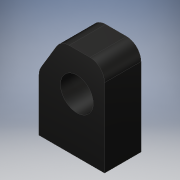
# Autodesk Inventor part: PilierCentral
Saved by Autodesk Inventor 2019 (Build 230136000, 136)
## iProperties
Created: 2019-07-30
Part Number: PilierCentral
Material: Plastique ABS
Document SubType Name: Modeling
Designer: Sébastien DI MERCURIO
Mass: 4.5474 g
Surface Area: 16.8462 cm^2
Volume: 4.29 cm^3
Density: 1.06 g/cm^3
Appearance: Lustré - Noir
Author: Sébastien DI MERCURIO
Autodesk Inventor part; units mm, degrees
ref_plane "YZ Plane" through (0, 0, 0) normal (1, 0, 0) x (0, 1, 0)
ref_plane "XZ Plane" through (0, 0, 0) normal (0, 1, 0) x (-1, 0, 0)
ref_plane "XY Plane" through (0, 0, 0) normal (0, 0, 1) x (1, 0, 0)
sketch "Esquisse1" plane through (0, 0, 0) normal (0, 0, 1) x (1, 0, 0)
  line L0 (0, 0) -> (0, 25.5)
  line L1 (0, 25.5) -> (-12, 25.5)
  line L2 (-12, 25.5) -> (-18, 15.5)
  line L3 (-18, 15.5) -> (-18, 0)
  line L4 (-18, 0) -> (0, 0)
  dimension "d0" = 18
  dimension "d1" = 25.5
  dimension "d2" = 15.5
  dimension "d3" = 12
  constraints: 10 end point, 2 perpendicular, 1 parallel, 1 vertical
  measures "d0" distance between parallel lines of L0 L3
  measures "d1" distance between parallel lines of L4 L1
  measures "d2" distance of L3.end L2.end
  measures "d3" distance of L0.end L1.end
extrude "Extrusion1" add sketch "Esquisse1" along normal blind 10
sketch "Esquisse2" plane through (0, 0, 10) normal (0, 0, 1) x (1, 0, 0)
  circle A0 centre (-7.6, 15) radius 4.5
  line L0 (-18, 0) -> (0, 0) projected
  line L1 (0, 0) -> (0, 25.5) projected
  dimension "d6" = 9
  dimension "d7" = 15
  dimension "d8" = 7.6
  constraints: 1 centre point
  measures "d6" diameter of A0
  measures "d7" distance from line of L0 A0.centre
  measures "d8" distance from line of L1 A0.centre
extrude "Extrusion2" cut sketch "Esquisse2" against normal through all
sketch "Esquisse3" plane through (-18, 0, 0) normal (-1, 0, 0) x (0, 0, 1)
  circle A0 centre (5, 10.5) radius 1.5
  circle A1 centre (5, 3.5) radius 1.5
  line L0 (10, 15.5) -> (10, 0) projected
  line L1 (0, 15.5) -> (0, 0) projected
  line L2 (0, 0) -> (10, 0) projected
  dimension "d11" = 3
  dimension "d12" = 10
  dimension "d13" = 5
  dimension "d14" = 7
  dimension "d15" = 3.5
  constraints: 2 centre point, 1 equal radius, 1 vertical alignment
  measures "d11" diameter of A0
  measures "d12" distance from line of L0 L1.end
  measures "d13" distance from line of L1 A1.centre
  measures "d14" distance of A1.centre A0.centre
  measures "d15" distance from line of L2 A1.centre
extrude "Extrusion3" cut sketch "Esquisse3" against normal blind 5
sketch "Esquisse4" plane through (-18, 0, 0) normal (0, -1, 0) x (1, 0, 0)
  circle A0 centre (8, 5) radius 1.5
  circle A1 centre (15, 5) radius 1.5
  line L0 (0, 10) -> (18, 10) projected
  line L1 (0, 0) -> (18, 0) projected
  line L2 (18, 0) -> (18, 10) projected
  dimension "d18" = 10
  dimension "d19" = 5
  dimension "d20" = 7
  dimension "d21" = 3
  dimension "d22" = 3
  constraints: 2 centre point, 1 equal radius, 1 horizontal alignment
  measures "d18" distance between parallel lines of L0 L1
  measures "d19" distance from line of L1 A0.centre
  measures "d20" distance of A1.centre A0.centre
  measures "d21" diameter of A0
  measures "d22" distance from line of L2 A1.centre
extrude "Extrusion4" cut sketch "Esquisse4" against normal blind 5
fillet "Congé1" radius 4 3 edges at (-12, 25.5, 5) (0, 25.5, 5) (-18, 15.5, 5)
equation "\"d13\" = 0.5 * d12"
equation "\"d19\" = 0.5 * d18"
